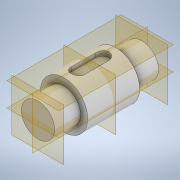
# Autodesk Inventor part: shaft1
Saved by Autodesk Inventor 2022 (Build 260153000, 153)
## iProperties
Created: 2023-12-21
Part Number: shaft1
Material: 一般
Document SubType Name: Modeling
Designer: ktamu
Density: 1 g/cm^3
Appearance: 既定
Author: ktamu
Autodesk Inventor part; units mm, degrees
sketch "スケッチ1" plane through (0, 0, 0) normal (0, 0, 1) x (1, 0, 0)
  circle A0 centre (0, 0) radius 17.5
  dimension "d0" = 35
  constraints: 1 centre point, 1 coincident
  measures "d0" diameter of A0
extrude "押し出し1" add sketch "スケッチ1" along normal blind 27.5
sketch "スケッチ2" plane through (0, 0, 27.5) normal (0, 0, 1) x (1, 0, 0)
  circle A0 centre (0, 0) radius 25
  dimension "d3" = 50
  constraints: 1 centre point, 1 coincident
  measures "d3" diameter of A0
extrude "押し出し2" add sketch "スケッチ2" along normal blind 55
sketch "スケッチ3" plane through (0, 0, 82.5) normal (0, 0, 1) x (1, 0, 0)
  circle A0 centre (0, 0) radius 17.5
  dimension "d6" = 35
  constraints: 1 centre point, 1 coincident
  measures "d6" diameter of A0
extrude "押し出し3" add sketch "スケッチ3" along normal blind 27.5
sketch "スケッチ4" plane through (0, 0, 0) normal (1, 0, 0) x (0, 1, 0)
  point P0 (0, 0)
ref_plane "作業平面2" through (0, 0, 55) normal (0, 0, 1) x (1, 0, 0)
ref_plane "作業平面1" through (0, 0, 110) normal (0, 0, 1) x (1, 0, 0)
ref_plane "作業平面3" through (0, 25, 0) normal (0, 1, 0) x (-1, 0, 0)
sketch "スケッチ8" plane through (0, 25, 0) normal (0, 1, 0) x (-1, 0, 0)
  line L0 (-7, 35) -> (7, 35)
  line L1 (0, 35) -> (0, 42)
  line L2 (0, 35) -> (7, 35) construction
  line L3 (-7, 35) -> (-7, 75)
  arc A0 (-7, 42) -> (7, 42) centre (0, 42) ccw
  line L4 (7, 75) -> (7, 35)
  line L5 (7, 42) -> (7, 35)
  line L6 (7, 35) -> (0, 35)
  line L7 (-7, 35) -> (-7, 42)
  line L8 (0, 35) -> (-7, 35)
  line L9 (7, 75) -> (-7, 75)
  line L10 (7, 55) -> (-7, 55)
  arc A1 (7, 68) -> (-7, 68) centre (0, 68) ccw
  point P0 (0, 0)
  dimension "d17" = 7
  dimension "d18" = 90
  dimension "d21" = 20
  constraints: 22 end point, 4 point on circle, 3 midpoint, 3 symmetric about line, 2 centre point, 1 coincident, 1 perpendicular, 1 point on line, 1 other
  measures "d17" distance of L1.start L1.end
  measures "d18" angle of L2 L1
  measures "d21" distance between parallel lines of L10 L9
extrude "押し出し5" cut sketch "スケッチ8" against normal blind 5.5 contours A0 L3 L10 L4 | L3 A1 L4 L10
